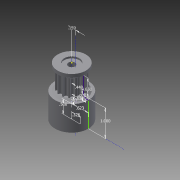
# Autodesk Inventor part: desno-gates-15
Saved by Autodesk Inventor 2015 (Build 190159000, 159)
## iProperties
Created: 2015-02-04
Part Number: desno-gates-15
Material: Generic
Document SubType Name: Modeling
Designer: sethbattis
Density: 1 g/cm^3
Appearance: Default
Author: sethbattis
Autodesk Inventor part; units mm, degrees
ref_plane "YZ Plane" through (0, 0, 0) normal (1, 0, 0) x (0, 1, 0)
ref_plane "XZ Plane" through (0, 0, 0) normal (0, 1, 0) x (-1, 0, 0)
ref_plane "XY Plane" through (0, 0, 0) normal (0, 0, 1) x (1, 0, 0)
sketch "Sketch1" plane through (0, 0, 0) normal (0, 0, 1) x (1, 0, 0)
  line L0 (0, 0) -> (0, 50.8) construction
  line L1 (0, 0) -> (50.8, 0) construction
  line L2 (0, 9.5479) -> (15.8115, 9.5479) construction
  line L3 (0, 0) -> (8.2867, 0) construction
  line L4 (8.2867, 0) -> (15.875, 0)
  line L5 (8.2867, 0) -> (8.2867, 12.7)
  line L6 (4.0259, 71.0633) -> (4.0259, -11.3243) construction
  line L7 (8.2867, 12.7) -> (4.0259, 12.7)
  line L8 (4.0259, 19.1008) -> (4.0259, 12.7)
  line L9 (4.0259, 19.1008) -> (0, 19.1008)
  line L10 (0, 41.91) -> (0, 19.1008)
  line L11 (11.3665, 41.91) -> (11.3665, 25.4)
  line L12 (11.3665, 25.4) -> (13.462, 23.622)
  line L13 (13.462, 23.622) -> (15.875, 23.622)
  line L14 (15.875, 23.622) -> (15.875, 0)
  line L15 (11.3665, 41.91) -> (0, 41.91)
  dimension "d12" = 15.8115
  dimension "d15" = 8.2867
  dimension "d55" = 4.0259
  dimension "d56" = 12.7
  dimension "d95" = 6.4008
  dimension "d97" = 16.51
  dimension "d99" = 1.778
  dimension "d100" = 11.3665
  dimension "d101" = 25.4
  dimension "d142" = 13.462
  constraints: 34 end point, 6 point on line, 5 perpendicular, 4 horizontal, 3 collinear, 1 vertical
  measures "d12" distance of L2.start L2.end
  measures "d15" distance of L3.start L3.end
  measures "d55" distance between parallel lines of L0 L6
  measures "d56" distance of L3.end L5.end
  measures "d95" distance of L8.start L7.end
  measures "d97" distance of L11.start L11.end
  measures "d99" vertical distance of L12.end L11.end
  measures "d100" distance between parallel lines of L10 L11
  measures "d101" distance from line of L4 L11.end
  measures "d142" distance from line of L10 L12.end
revolve "Revolution1" add sketch "Sketch1" angle 360 about axis through (0, 0, 0) along (0, 1, 0)
sketch "Sketch2" plane through (0, 0, 0) normal (0, -1, 0) x (1, 0, 0)
  circle A0 centre (0, 0) radius 8.2867 construction
  line L0 (-2.2055, 7.9879) -> (-2.2121, 9.8928)
  circle A1 centre (0, 0) radius 10.1371 construction
  line L1 (2.1506, 8.0028) -> (2.144, 9.9078)
  line L2 (-2.2055, 7.9879) -> (2.1506, 8.0028) construction
  arc A2 (2.144, 9.9078) -> (-2.2121, 9.8928) centre (0, 0) ccw
  arc A3 (2.1506, 8.0028) -> (-2.2055, 7.9879) centre (0, 0) ccw
  dimension "d43" = 1.905
  dimension "d44" = 4.3561
  constraints: 8 point on circle, 6 end point, 3 centre point, 2 coincident, 1 concentric, 1 parallel, 1 perpendicular
  measures "d43" distance of L0.start L0.end
  measures "d44" distance of L0.start L1.start
extrude "Extrusion1" cut sketch "Sketch2" against normal blind 12.7
pattern_circular "Circular Pattern2" count 6 over 360 about axis through (0, 6.35, 0) along (0, -1, 0) of "Extrusion1"
sketch "Sketch12" plane through (0, 41.91, 0) normal (0, 1, 0) x (1, 0, 0)
  circle A0 centre (0, 0) radius 11.3665 construction
  circle A1 centre (0, 0) radius 9.2837 construction
  circle A2 centre (0, 0) radius 4.0259 projected
  line L0 (0, 0) -> (0, 13.462) construction
  circle A3 centre (0, 0) radius 13.462 projected
  line L1 (0, 0) -> (-1.9302, 9.0808) construction
  line L2 (0, 0) -> (0, 0) construction
  circle A4 centre (-2.2602, 10.6332) radius 1.5871 construction
  circle A5 centre (2.2602, 10.6332) radius 1.5871 construction
  line L3 (-0.6731, 11.3665) -> (0.6731, 11.3665)
  line L4 (0.6731, 11.3665) -> (0.6731, 10.6332)
  arc A6 (0.6731, 10.6332) -> (3.71, 9.9877) centre (2.2602, 10.6332) ccw
  line L5 (4.0083, 10.6576) -> (5.2381, 10.11)
  line L6 (4.0083, 10.6576) -> (3.71, 9.9877)
  line L7 (-0.6731, 11.3665) -> (-0.6731, 9.2593) construction
  arc A7 (4.0083, 10.6576) -> (0.6731, 11.3665) centre (0.9935, 4.674) ccw
  dimension "d152" = 22.733
  dimension "d153" = 18.5674
  dimension "d154" = 24
  dimension "d155" = 1.3462
  dimension "d156" = 24
  constraints: 16 end point, 8 point on circle, 6 centre point, 6 tangent, 4 coincident, 3 vertical, 2 line through centre, 1 equal length, 1 equal radius, 1 horizontal, 1 midpoint, 1 perpendicular, 1 symmetric about line, 1 vertical alignment, 2 other
  measures "d152" diameter of A0
  measures "d153" diameter of A1
  measures "d154" angle of L2 L1
  measures "d155" distance of L3.start L3.end
  measures "d156" angle of L6 L4
extrude "Extrusion6" cut sketch "Sketch12" against normal blind 16.51 contours A7 L6 A6 L4
fillet "Fillet8" radius 0.127 2 edges at (0.6731, 33.655, -11.3466) (4.0002, 33.655, -10.6394)
pattern_circular "Circular Pattern4" count 15 over 360 about axis through (0, 33.655, 0) along (0, -1, 0) of "Extrusion6", "Fillet8"
sketch "Sketch14" plane through (0, 0, 0) normal (0, 0, 1) x (1, 0, 0)
  line L0 (0, 41.91) -> (11.3665, 41.91)
  line L1 (11.3665, 41.91) -> (13.462, 43.688)
  line L2 (13.462, 43.688) -> (13.462, 46.863)
  line L3 (13.462, 46.863) -> (0, 46.863)
  line L4 (0, 46.863) -> (0, 41.91)
  point P0 (0, 0)
  point P1 (13.462, 45.2755)
  dimension "d166" = 11.3665
  dimension "d167" = 1.778
  dimension "d168" = 13.462
  dimension "d169" = 3.175
  dimension "d181" = 4.953
  dimension "d182" = 2.0955
  constraints: 10 end point, 2 horizontal, 1 midpoint, 1 parallel, 1 perpendicular
  measures "d166" distance of L0.start L0.end
  measures "d167" vertical distance of L1.end L0.end
  measures "d168" distance between parallel lines of L2 L4
  measures "d169" distance of L1.end L2.end
  measures "d181" distance of L3.end L0.start
  measures "d182" horizontal distance of L1.end L0.end
revolve "Revolution2" add sketch "Sketch14" angle 360 about axis through (0, 46.863, 0) along (0, -1, 0)
sketch "Sketch16" plane through (0, 12.7, 0) normal (0, -1, 0) x (0.9999941, 0, 0.0034377)
  circle A0 centre (0, 0) radius 6.4135 construction
  line L0 (5.5543, 3.2067) -> (5.5543, -3.2068)
  line L1 (5.5543, -3.2068) -> (0, -6.4135)
  line L2 (0, -6.4135) -> (-5.5543, -3.2068)
  line L3 (-5.5543, -3.2068) -> (-5.5543, 3.2067)
  line L4 (-5.5543, 3.2067) -> (0, 6.4135)
  line L5 (5.5543, 3.2067) -> (0, 6.4135)
  dimension "d172" = 12.827
  constraints: 12 end point, 6 point on circle, 3 equal length, 2 parallel, 2 vertical, 1 centre point, 1 coincident
  measures "d172" diameter of A0
extrude "Extrusion7" cut sketch "Sketch16" against normal blind 10.7442
sketch "Sketch17" plane through (0, 23.4442, 0) normal (0, -1, 0) x (0.9999941, 0, 0.0034377)
  circle A0 centre (0, 0) radius 3.175
  dimension "d175" = 6.35
  constraints: 1 centre point, 1 coincident
  measures "d175" diameter of A0
extrude "Extrusion8" cut sketch "Sketch17" against normal through all
sketch "Sketch18" plane through (0, 46.863, 0) normal (0, 1, 0) x (1, 0, 0)
  point P0 (0, 0)
sketch "Sketch19" plane through (0, 46.863, 0) normal (0, 1, 0) x (1, 0, 0)
  circle A0 centre (0, 0) radius 7.2009
  dimension "d178" = 14.4018
  constraints: 1 centre point, 1 coincident
  measures "d178" diameter of A0
extrude "Extrusion9" cut sketch "Sketch19" against normal blind 1.6002
body "Solid1"
